lead-screw to upper base connector_v3 (Autodesk Fusion 360 design; units mm, degrees)
Autodesk Fusion 360 part; units mm, degrees
sketch "Sketch1" plane through (0, 0, 0) normal (0, 1, 0) x (1, 0, 0)
  line L0 (0, 0) -> (40, 0)
  line L1 (40, 0) -> (40, -70)
  line L2 (40, -70) -> (0, -70)
  line L3 (0, -70) -> (0, 0)
  circle A0 centre (20, -15) radius 5
  circle A1 centre (20, -15) radius 11
  circle A2 centre (14.5, -20.5) radius 1.5
  circle A3 centre (25.5, -20.5) radius 1.5
  circle A4 centre (14.5, -9.5) radius 1.5
  circle A5 centre (25.5, -9.5) radius 1.5
  line L4 (20, -20) -> (20, -67) construction
  line L5 (0, -57) -> (40, -57) construction
  line L6 (20, -20) -> (20, -15) construction
  point P0 (20, -15)
  dimension "d1" = 40
  dimension "d2" = 70
  dimension "d3" = 10
  dimension "d4" = 15
  dimension "d5" = 22
  dimension "d6" = 11
  dimension "d7" = 11
  dimension "d8" = 3
  dimension "d9" = 3
  dimension "d10" = 3
  dimension "d11" = 3
  dimension "d12" = 52
  dimension "d13" = 42
  constraint horizontal L0
  constraint vertical L1
  constraint horizontal L2
  constraint vertical L3
  constraint coincident L0.start L3.end
  constraint concentric A0 A1
  constraint coincident P0 A0.centre
  constraint vertical L4
  constraint coincident L3 L5.start
  constraint coincident L1 L5.end
  constraint perpendicular L1 L5
  constraint coincident A0 L4.start
  constraint parallel L4 L6
  measures "d1" distance of L0.start L0.end
  measures "d2" distance of L0.start L2.end
  measures "d3" diameter of A0
  measures "d4" distance of L0 P0
  measures "d5" diameter of A1
  measures "d6" distance of A2.centre A3.centre
  measures "d7" distance of A2.centre A4.centre
  measures "d8" diameter of A2
  measures "d9" diameter of A3
  measures "d10" diameter of A4
  measures "d11" diameter of A5
  measures "d12" distance of P0 L4.end
  measures "d13" distance of P0 L5
extrude "Extrude1" add sketch "Sketch1" along normal blind 25 contours L0 L1 L2 L3 | A1 | A2 | A3 | A4 | A5
extrude "Extrude2" cut sketch "Sketch1" along normal blind 4 contours A1
extrude "Extrude3" cut sketch "Sketch1" along normal blind 27 contours A2 | A3 | A4 | A5
